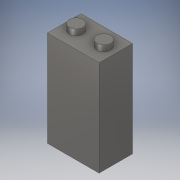
# Autodesk Inventor part: 9VBatterie_2017only
Saved by Autodesk Inventor 2017 (Build 210142000, 142)
## iProperties
Part Number: 9VBatterie_2017only
Material: Edelstahl
Document SubType Name: Modeling
Designer: Youri
Density: 8 g/cm^3
Appearance: Halbpoliert
Mass: 174.662 g
Surface Area: 52.1315 cm^2
Volume: 21.8328 cm^3
Author: Youri
Autodesk Inventor part; units mm, degrees
ref_plane "YZ Plane" through (0, 0, 0) normal (1, 0, 0) x (0, 1, 0)
ref_plane "XZ Plane" through (0, 0, 0) normal (0, 1, 0) x (-1, 0, 0)
ref_plane "XY Plane" through (0, 0, 0) normal (0, 0, 1) x (1, 0, 0)
sketch "Skizze1" plane through (0, 0, 0) normal (0, 1, 0) x (-1, 0, 0)
  line L0 (24.1361, 0) -> (-12.5439, 0) projected
  line L1 (0, -33.95) -> (0, 33.95) projected
  line L2 (-7.3039, 24.25) -> (18.8961, 24.25)
  line L3 (18.8961, 24.25) -> (18.8961, -24.25)
  line L4 (18.8961, -24.25) -> (-7.3039, -24.25)
  line L5 (-7.3039, -24.25) -> (-7.3039, 24.25)
  point P0 (0, 0)
  dimension "d0" = 48.5
  dimension "d1" = 26.2
  constraints: 8 end point, 2 parallel, 1 horizontal, 1 perpendicular, 1 other
  measures "d0" distance of L2.end L3.end
  measures "d1" distance of L2.start L2.end
extrude "Extrusion1" add sketch "Skizze1" along normal blind 17
sketch "Skizze3" plane through (-18.8961, 0, 24.25) normal (0, 0, 1) x (1, 0, 0)
  line L0 (26.2, 0) -> (0, 0) projected
  line L1 (0, 0) -> (0, 17) projected
  line L2 (0, 17) -> (26.2, 17) projected
  line L3 (13.1, 17) -> (13.1, 0)
  circle A0 centre (6.1, 8.5) radius 3.5
  circle A1 centre (20.1, 8.5) radius 3.5
  point P0 (18.8961, 0)
  dimension "d7" = 13.1
  dimension "d8" = 7
  dimension "d9" = 8.5
  dimension "d10" = 7
  constraints: 2 centre point, 2 end point, 2 midpoint, 1 perpendicular, 1 symmetric about line, 1 other
  measures "d7" distance between parallel lines of L3 L1
  measures "d8" distance from line of L3 A0.centre
  measures "d9" distance from line of L0 A0.centre
  measures "d10" diameter of A0
extrude "Extrusion2" add sketch "Skizze3" along normal blind 3 contours A0 | A1
equation "\"d10\" = usedParameter"
equation "\"usedParameter\" = 7"
equation "\"unusedParameter\" = 42"
